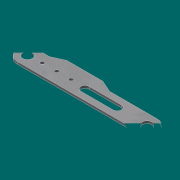
# Autodesk Inventor part: rinnku
Saved by Autodesk Inventor 2016 (Build 200138000, 138)
## iProperties
Created: 2016-08-23
Part Number: rinnku
Material: GFRP
Document SubType Name: Modeling
Designer: hiro
Density: 1.75 g/cm^3
Appearance: 滑らか - 淡い灰色
Mass: 6.14531 g
Surface Area: 43.3352 cm^2
Volume: 3.5116 cm^3
Author: hiro
Autodesk Inventor part; units mm, degrees
ref_plane "YZ Plane" through (0, 0, 0) normal (1, 0, 0) x (0, 1, 0)
ref_plane "XZ Plane" through (0, 0, 0) normal (0, 1, 0) x (-1, 0, 0)
ref_plane "XY Plane" through (0, 0, 0) normal (0, 0, 1) x (1, 0, 0)
sketch "スケッチ1" plane through (0, 0, 0) normal (0, 0, 1) x (1, 0, 0)
  line L0 (-50, 0) -> (50, 0) construction
  circle A0 centre (-50, 0) radius 4.05
  circle A1 centre (50, 0) radius 4.05
  line L1 (-50, 8.5) -> (43, 8.5)
  line L2 (-50, -8.5) -> (43, -8.5)
  arc A2 (-50, 8.5) -> (-50, -8.5) centre (-50, 0) ccw
  arc A3 (25.013, -3.45) -> (25.013, 3.45) centre (25.013, 0) ccw
  line L3 (25.013, -3.45) -> (-2, -3.45)
  line L4 (25.013, 3.45) -> (-2, 3.45)
  arc A4 (-2, 3.45) -> (-2, -3.45) centre (-2, 0) ccw
  line L5 (43, -8.5) -> (50.0601, -8.4498)
  line L6 (43, 8.5) -> (50.0601, 8.4498)
  arc A5 (50.0601, -8.4498) -> (50.0601, 8.4498) centre (50, 0) ccw
  line L7 (-41, -8.5) -> (-12, -8.5) construction
  line L8 (-12, -8.5) -> (-12, -3.5) construction
  line L9 (-12, -3.5) -> (-41, -3.5) construction
  line L10 (-41, -3.5) -> (-41, -8.5) construction
  line L11 (-41, -6) -> (-12, -6) construction
  circle A6 centre (-26.5, -6) radius 1.55
  circle A7 centre (-38.5, -6) radius 1.55
  circle A8 centre (-14.5, -6) radius 1.55
  line L12 (-26.5, -6) -> (-26.5, -3.5) construction
  line L13 (0, 13) -> (-30, 13)
  line L14 (-30, 13) -> (-40, 8.5)
  line L15 (0, 13) -> (10, 8.5)
  point P0 (0, 0)
  point P1 (0, 0)
  dimension "d0" = 100
  dimension "d1" = 8.1
  dimension "d2" = 8.5
  dimension "d5" = 3.45
  dimension "d7" = 52
  dimension "d8" = 8.1
  dimension "d9" = 7
  dimension "d10" = 8.45
  dimension "d11" = 27.013
  dimension "d12" = 5
  dimension "d13" = 29
  dimension "d14" = 3.1
  dimension "d15" = 2.5
  dimension "d16" = 9
  dimension "d17" = 13
  dimension "d19" = 10
  dimension "d20" = 30
  dimension "d22" = 10
  dimension "d23" = 40
  dimension "d24" = 0
  constraints: 32 end point, 9 centre point, 8 point on circle, 8 tangent, 6 horizontal, 5 midpoint, 4 coincident, 4 point on line, 2 equal radius, 2 horizontal alignment, 2 parallel, 1 perpendicular, 1 symmetric about line, 1 vertical alignment
  measures "d0" distance of L0.start L0.end
  measures "d1" diameter of A0
  measures "d2" radius of A2
  measures "d5" radius of A3
  measures "d7" distance of L0.end A4.centre
  measures "d8" diameter of A1
  measures "d9" horizontal distance of L1.end L0.end
  measures "d10" radius of A5
  measures "d11" distance of A4.centre A3.centre
  measures "d12" distance of L9.end L7.start
  measures "d13" distance of L8.end L9.end
  measures "d14" diameter of A6
  measures "d15" distance from line of L10 A7.centre
  measures "d16" distance from line of L10 L0.start
  measures "d17" distance from line of L0.end L13
  measures "d19" horizontal distance of L14.end L13.end
  measures "d20" distance of L13.start L13.end
  measures "d22" horizontal distance of L15.end L13.start
  measures "d23" horizontal distance of L0.end L15.end
  measures "d24" distance between parallel lines of L2 L7
extrude "押し出し1" add sketch "スケッチ1" along normal blind 2
fillet "フィレット1" radius 2 4 edges at (-40, 8.5, 1) (-30, 13, 1) (0, 13, 1) (43, 8.5, 1)
equation "\"d7\" = 2 * d28"
equation "\"d8\" = d1"
equation "\"d11\" = d39"
equation "\"d19\" = d18"
equation "\"d22\" = d19"
equation "\"d28\" = 26"
equation "\"d39\" = 27.012989"
equation "\"d18\" = 10"
